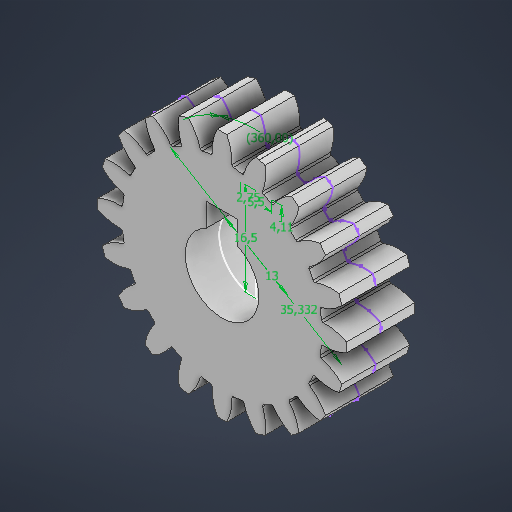
# Autodesk Inventor part: Engrenagem 2
Saved by Autodesk Inventor 2026.2 (Build 302298000, 298)
## iProperties
Created: 2026-09-11
Part Number: Engrenagem 2
Material: Genérico
Document SubType Name: Modeling
Designer: IFSP
Density: 1 g/cm^3
Appearance: Padrão
Author: IFSP
Autodesk Inventor part; units mm, degrees
ref_plane "YZ Plane" through (0, 0, 0) normal (1, 0, 0) x (0, 1, 0)
ref_plane "XZ Plane" through (0, 0, 0) normal (0, 1, 0) x (-1, 0, 0)
ref_plane "XY Plane" through (0, 0, 0) normal (0, 0, 1) x (1, 0, 0)
sketch "Esboço1" plane through (0, 0, 0) normal (0, 0, 1) x (1, 0, 0)
  circle A0 centre (0, 0) radius 6.5
  line L0 (0, -6.5) -> (0, 10)
  line L1 (0, 10) -> (-2.75, 10)
  line L2 (-2.75, 10) -> (2.75, 10)
  line L3 (-2.75, 10) -> (-2.75, 5.8896)
  line L4 (2.75, 10) -> (2.75, 5.8896)
  arc A1 (-2.0125, 17.551) -> (2.0125, 17.551) centre (0, 0) ccw
  line L5 (-1.57, 19.9383) -> (-1.5695, 19.9383)
  line L6 (0, 0) -> (0, 22)
  line L7 (6.5635, 20.9981) -> (6.5635, 20.9805)
  arc A2 (6.563, 18.8925) -> (6.5635, 18.896) centre (-1.57, 19.9383) ccw
  arc A3 (6.5635, 20.9805) -> (6.5611, 20.9988) centre (-1.57, 19.9383) ccw
  line L8 (6.5635, 18.896) -> (6.5635, 18.8923)
  arc A4 (6.5635, 20.9842) -> (6.5616, 20.9987) centre (-1.5695, 19.9383) ccw
  arc A5 (-0.8328, 21.9842) -> (-1.7469, 17.8617) centre (6.4458, 18.2077) ccw
  arc A6 (0.9393, 12.1317) -> (0.9394, 12.1315) centre (6.4458, 18.2077) ccw
  line L9 (-1.57, 0) -> (-1.57, 10)
  line L10 (-1.57, 19.9361) -> (-1.57, 19.9383)
  arc A7 (-2.0125, 17.551) -> (-1.7469, 17.8617) centre (-2.0466, 17.849) ccw
  arc A8 (1.7469, 17.8617) -> (0.8328, 21.9842) centre (-6.4458, 18.2077) ccw
  arc A9 (1.7469, 17.8617) -> (2.0125, 17.551) centre (2.0466, 17.849) ccw
  arc A10 (6.5635, 20.9981) -> (6.5611, 20.9988) centre (0, 0) ccw
  arc A11 (0.8328, 21.9842) -> (-0.8328, 21.9842) centre (0, 0) ccw
  circle A12 centre (0, 0) radius 17.666
  arc A13 (-3.8582, 17.5273) -> (-6.0014, 21.1656) centre (-11.7568, 15.3247) ccw
  arc A14 (-6.0014, 21.1656) -> (-7.5856, 20.6509) centre (0, 0) ccw
  arc A15 (-7.5856, 20.6509) -> (-7.181, 16.4477) centre (0.5038, 19.3084) ccw
  arc A16 (-7.3375, 16.0701) -> (-7.181, 16.4477) centre (-7.4621, 16.343) ccw
  arc A17 (-3.8582, 17.5273) -> (-3.5096, 17.3139) centre (-3.5692, 17.6079) ccw
  arc A18 (-9.0856, 15.4772) -> (-12.2482, 18.2751) centre (-15.917, 10.9416) ccw
  arc A19 (-12.2482, 18.2751) -> (-13.5958, 17.2961) centre (0, 0) ccw
  arc A20 (-13.5958, 17.2961) -> (-11.9121, 13.4236) centre (-5.4875, 18.5191) ccw
  arc A21 (-11.9443, 13.0162) -> (-11.9121, 13.4236) centre (-12.1472, 13.2372) ccw
  arc A22 (-9.0856, 15.4772) -> (-8.6881, 15.382) centre (-8.8356, 15.6432) ccw
  arc A23 (-13.4236, 11.9121) -> (-17.2961, 13.5958) centre (-18.5191, 5.4875) ccw
  arc A24 (-17.2961, 13.5958) -> (-18.2751, 12.2482) centre (0, 0) ccw
  arc A25 (-18.2751, 12.2482) -> (-15.4772, 9.0856) centre (-10.9416, 15.917) ccw
  arc A26 (-15.382, 8.6881) -> (-15.4772, 9.0856) centre (-15.6432, 8.8356) ccw
  arc A27 (-13.4236, 11.9121) -> (-13.0162, 11.9443) centre (-13.2372, 12.1472) ccw
  arc A28 (-16.4477, 7.181) -> (-20.6509, 7.5856) centre (-19.3084, -0.5038) ccw
  arc A29 (-20.6509, 7.5856) -> (-21.1656, 6.0014) centre (0, 0) ccw
  arc A30 (-21.1656, 6.0014) -> (-17.5273, 3.8582) centre (-15.3247, 11.7568) ccw
  arc A31 (-17.3139, 3.5096) -> (-17.5273, 3.8582) centre (-17.6079, 3.5692) ccw
  arc A32 (-16.4477, 7.181) -> (-16.0701, 7.3375) centre (-16.343, 7.4621) ccw
  arc A33 (-17.8617, 1.7469) -> (-21.9842, 0.8328) centre (-18.2077, -6.4458) ccw
  arc A34 (-21.9842, 0.8328) -> (-21.9842, -0.8328) centre (0, 0) ccw
  arc A35 (-21.9842, -0.8328) -> (-17.8617, -1.7469) centre (-18.2077, 6.4458) ccw
  arc A36 (-17.551, -2.0125) -> (-17.8617, -1.7469) centre (-17.849, -2.0466) ccw
  arc A37 (-17.8617, 1.7469) -> (-17.551, 2.0125) centre (-17.849, 2.0466) ccw
  arc A38 (-17.5273, -3.8582) -> (-21.1656, -6.0014) centre (-15.3247, -11.7568) ccw
  arc A39 (-21.1656, -6.0014) -> (-20.6509, -7.5856) centre (0, 0) ccw
  arc A40 (-20.6509, -7.5856) -> (-16.4477, -7.181) centre (-19.3084, 0.5038) ccw
  arc A41 (-16.0701, -7.3375) -> (-16.4477, -7.181) centre (-16.343, -7.4621) ccw
  arc A42 (-17.5273, -3.8582) -> (-17.3139, -3.5096) centre (-17.6079, -3.5692) ccw
  arc A43 (-15.4772, -9.0856) -> (-18.2751, -12.2482) centre (-10.9416, -15.917) ccw
  arc A44 (-18.2751, -12.2482) -> (-17.2961, -13.5958) centre (0, 0) ccw
  arc A45 (-17.2961, -13.5958) -> (-13.4236, -11.9121) centre (-18.5191, -5.4875) ccw
  arc A46 (-13.0162, -11.9443) -> (-13.4236, -11.9121) centre (-13.2372, -12.1472) ccw
  arc A47 (-15.4772, -9.0856) -> (-15.382, -8.6881) centre (-15.6432, -8.8356) ccw
  arc A48 (-11.9121, -13.4236) -> (-13.5958, -17.2961) centre (-5.4875, -18.5191) ccw
  arc A49 (-13.5958, -17.2961) -> (-12.2482, -18.2751) centre (0, 0) ccw
  arc A50 (-12.2482, -18.2751) -> (-9.0856, -15.4772) centre (-15.917, -10.9416) ccw
  arc A51 (-8.6881, -15.382) -> (-9.0856, -15.4772) centre (-8.8356, -15.6432) ccw
  arc A52 (-11.9121, -13.4236) -> (-11.9443, -13.0162) centre (-12.1472, -13.2372) ccw
  arc A53 (-7.181, -16.4477) -> (-7.5856, -20.6509) centre (0.5038, -19.3084) ccw
  arc A54 (-7.5856, -20.6509) -> (-6.0014, -21.1656) centre (0, 0) ccw
  arc A55 (-6.0014, -21.1656) -> (-3.8582, -17.5273) centre (-11.7568, -15.3247) ccw
  arc A56 (-3.5096, -17.3139) -> (-3.8582, -17.5273) centre (-3.5692, -17.6079) ccw
  arc A57 (-7.181, -16.4477) -> (-7.3375, -16.0701) centre (-7.4621, -16.343) ccw
  arc A58 (-1.7469, -17.8617) -> (-0.8328, -21.9842) centre (6.4458, -18.2077) ccw
  arc A59 (-0.8328, -21.9842) -> (0.8328, -21.9842) centre (0, 0) ccw
  arc A60 (0.8328, -21.9842) -> (1.7469, -17.8617) centre (-6.4458, -18.2077) ccw
  arc A61 (2.0125, -17.551) -> (1.7469, -17.8617) centre (2.0466, -17.849) ccw
  arc A62 (-1.7469, -17.8617) -> (-2.0125, -17.551) centre (-2.0466, -17.849) ccw
  arc A63 (3.8582, -17.5273) -> (6.0014, -21.1656) centre (11.7568, -15.3247) ccw
  arc A64 (6.0014, -21.1656) -> (7.5856, -20.6509) centre (0, 0) ccw
  arc A65 (7.5856, -20.6509) -> (7.181, -16.4477) centre (-0.5038, -19.3084) ccw
  arc A66 (7.3375, -16.0701) -> (7.181, -16.4477) centre (7.4621, -16.343) ccw
  arc A67 (3.8582, -17.5273) -> (3.5096, -17.3139) centre (3.5692, -17.6079) ccw
  arc A68 (9.0856, -15.4772) -> (12.2482, -18.2751) centre (15.917, -10.9416) ccw
  arc A69 (12.2482, -18.2751) -> (13.5958, -17.2961) centre (0, 0) ccw
  arc A70 (13.5958, -17.2961) -> (11.9121, -13.4236) centre (5.4875, -18.5191) ccw
  arc A71 (11.9443, -13.0162) -> (11.9121, -13.4236) centre (12.1472, -13.2372) ccw
  arc A72 (9.0856, -15.4772) -> (8.6881, -15.382) centre (8.8356, -15.6432) ccw
  arc A73 (13.4236, -11.9121) -> (17.2961, -13.5958) centre (18.5191, -5.4875) ccw
  arc A74 (17.2961, -13.5958) -> (18.2751, -12.2482) centre (0, 0) ccw
  arc A75 (18.2751, -12.2482) -> (15.4772, -9.0856) centre (10.9416, -15.917) ccw
  arc A76 (15.382, -8.6881) -> (15.4772, -9.0856) centre (15.6432, -8.8356) ccw
  arc A77 (13.4236, -11.9121) -> (13.0162, -11.9443) centre (13.2372, -12.1472) ccw
  arc A78 (16.4477, -7.181) -> (20.6509, -7.5856) centre (19.3084, 0.5038) ccw
  arc A79 (20.6509, -7.5856) -> (21.1656, -6.0014) centre (0, 0) ccw
  arc A80 (21.1656, -6.0014) -> (17.5273, -3.8582) centre (15.3247, -11.7568) ccw
  arc A81 (17.3139, -3.5096) -> (17.5273, -3.8582) centre (17.6079, -3.5692) ccw
  arc A82 (16.4477, -7.181) -> (16.0701, -7.3375) centre (16.343, -7.4621) ccw
  arc A83 (17.8617, -1.7469) -> (21.9842, -0.8328) centre (18.2077, 6.4458) ccw
  arc A84 (21.9842, -0.8328) -> (21.9842, 0.8328) centre (0, 0) ccw
  arc A85 (21.9842, 0.8328) -> (17.8617, 1.7469) centre (18.2077, -6.4458) ccw
  arc A86 (17.551, 2.0125) -> (17.8617, 1.7469) centre (17.849, 2.0466) ccw
  arc A87 (17.8617, -1.7469) -> (17.551, -2.0125) centre (17.849, -2.0466) ccw
  arc A88 (17.5273, 3.8582) -> (21.1656, 6.0014) centre (15.3247, 11.7568) ccw
  arc A89 (21.1656, 6.0014) -> (20.6509, 7.5856) centre (0, 0) ccw
  arc A90 (20.6509, 7.5856) -> (16.4477, 7.181) centre (19.3084, -0.5038) ccw
  arc A91 (16.0701, 7.3375) -> (16.4477, 7.181) centre (16.343, 7.4621) ccw
  arc A92 (17.5273, 3.8582) -> (17.3139, 3.5096) centre (17.6079, 3.5692) ccw
  arc A93 (15.4772, 9.0856) -> (18.2751, 12.2482) centre (10.9416, 15.917) ccw
  arc A94 (18.2751, 12.2482) -> (17.2961, 13.5958) centre (0, 0) ccw
  arc A95 (17.2961, 13.5958) -> (13.4236, 11.9121) centre (18.5191, 5.4875) ccw
  arc A96 (13.0162, 11.9443) -> (13.4236, 11.9121) centre (13.2372, 12.1472) ccw
  arc A97 (15.4772, 9.0856) -> (15.382, 8.6881) centre (15.6432, 8.8356) ccw
  arc A98 (11.9121, 13.4236) -> (13.5958, 17.2961) centre (5.4875, 18.5191) ccw
  arc A99 (13.5958, 17.2961) -> (12.2482, 18.2751) centre (0, 0) ccw
  arc A100 (12.2482, 18.2751) -> (9.0856, 15.4772) centre (15.917, 10.9416) ccw
  arc A101 (8.6881, 15.382) -> (9.0856, 15.4772) centre (8.8356, 15.6432) ccw
  arc A102 (11.9121, 13.4236) -> (11.9443, 13.0162) centre (12.1472, 13.2372) ccw
  arc A103 (7.181, 16.4477) -> (7.5856, 20.6509) centre (-0.5038, 19.3084) ccw
  arc A104 (7.5856, 20.6509) -> (6.0014, 21.1656) centre (0, 0) ccw
  arc A105 (6.0014, 21.1656) -> (3.8582, 17.5273) centre (11.7568, 15.3247) ccw
  arc A106 (3.5096, 17.3139) -> (3.8582, 17.5273) centre (3.5692, 17.6079) ccw
  arc A107 (7.181, 16.4477) -> (7.3375, 16.0701) centre (7.4621, 16.343) ccw
  point P0 (0, 10)
  point P1 (-6.7984, 20.9232)
  point P2 (-7.6537, 18.4752)
  point P3 (-12.9313, 17.7984)
  point P4 (-12.9883, 15.2058)
  point P5 (-17.7984, 12.9313)
  point P6 (-17.0515, 10.448)
  point P7 (-20.9232, 6.7984)
  point P8 (-19.4455, 4.6674)
  point P9 (-22, 0)
  point P10 (-19.9361, -1.57)
  point P11 (-20.9232, -6.7984)
  point P12 (-18.4752, -7.6537)
  point P13 (-17.7984, -12.9313)
  point P14 (-15.2058, -12.9883)
  point P15 (-12.9313, -17.7984)
  point P16 (-10.448, -17.0515)
  point P17 (-6.7984, -20.9232)
  point P18 (-4.6674, -19.4455)
  point P19 (0, -22)
  point P20 (1.57, -19.9361)
  point P21 (6.7984, -20.9232)
  point P22 (7.6537, -18.4752)
  point P23 (12.9313, -17.7984)
  point P24 (12.9883, -15.2058)
  point P25 (17.7984, -12.9313)
  point P26 (17.0515, -10.448)
  point P27 (20.9232, -6.7984)
  point P28 (19.4455, -4.6674)
  point P29 (22, 0)
  point P30 (19.9361, 1.57)
  point P31 (20.9232, 6.7984)
  point P32 (18.4752, 7.6537)
  point P33 (17.7984, 12.9313)
  point P34 (15.2058, 12.9883)
  point P35 (12.9313, 17.7984)
  point P36 (10.448, 17.0515)
  point P37 (6.7984, 20.9232)
  point P38 (4.6674, 19.4455)
  point P39 (-11.9443, 13.0162)
  point P40 (-8.6881, 15.382)
  point P41 (-15.382, 8.6881)
  point P42 (-13.0162, 11.9443)
  point P43 (-17.3139, 3.5096)
  point P44 (-16.0701, 7.3375)
  point P45 (-17.551, -2.0125)
  point P46 (-17.551, 2.0125)
  point P47 (-16.0701, -7.3375)
  point P48 (-15.382, -8.6881)
  point P49 (-8.6881, -15.382)
  point P50 (-7.3375, -16.0701)
  point P51 (-2.0125, -17.551)
  point P52 (7.3375, -16.0701)
  point P53 (8.6881, -15.382)
  point P54 (15.382, -8.6881)
  point P55 (16.0701, -7.3375)
  point P56 (17.551, 2.0125)
  point P57 (17.551, -2.0125)
  point P58 (16.0701, 7.3375)
  point P59 (15.382, 8.6881)
  point P60 (8.6881, 15.382)
  point P61 (11.9443, 13.0162)
  point P62 (6.5611, 20.9988)
  point P63 (3.5096, 17.3139)
  point P64 (-7.3375, 16.0701)
  dimension "d9" = 35.332
  dimension "d0" = 13
  dimension "d1" = 16.5
  dimension "d3" = 2.75
  dimension "d4" = 5.5
  dimension "d5" = 4.1104
  dimension "d23" = 360
  constraints: 275 point on circle, 106 centre point, 22 end point, 5 symmetric about line, 5 vertical, 4 coincident, 3 perpendicular, 3 point on line, 2 parallel, 1 tangent, 391 other
  measures "d0" diameter of A0
  measures "d1" distance of L0.start L0.end
  measures "d3" distance of L0.end L1.end
  measures "d4" distance of L1.end L2.end
  measures "d5" distance of L4.end L2.end
extrude "Extrusão1" add sketch "Esboço1" along normal mid plane 12 contours A6 A1 A12 | A6 A12 L6 | L6 A12 A1 A6 | A12 A6 A5 A11 L6 | L6 A11 A8 A9 A12 | A12 A7 A6
extrude "Extrusão2" add sketch "Esboço1" along normal mid plane 12 contours A96 A95 A94 A93 A97 A1 | A1 A101 A100 A99 A98 A102 | A106 A105 A104 A3 A103 A107 A1 | A1 A16 A15 A14 A13 A17 | A91 A90 A89 A88 A92 A1 | A1 A21 A20 A19 A18 A22 | A86 A85 A84 A83 A87 A1 | A1 A26 A25 A24 A23 A27 | A1 A31 A30 A29 A28 A32 | A81 A80 A79 A78 A82 A1 | A1 A36 A35 A34 A33 A37 | A76 A75 A74 A73 A77 A1 | A1 A41 A40 A39 A38 A42 | A71 A70 A69 A68 A72 A1 | A1 A46 A45 A44 A43 A47 | A66 A65 A64 A63 A67 A1 | A1 A51 A50 A49 A48 A52 | A61 A60 A59 A58 A62 A1 | A1 A56 A55 A54 A53 A57
